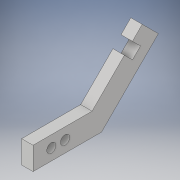
# Autodesk Inventor part: arm
Saved by Autodesk Inventor 2019 (Build 230136000, 136)
## iProperties
Created: 2018-09-08
Part Number: arm
Material: Generic
Document SubType Name: Modeling
Designer: mspet
Density: 1 g/cm^3
Appearance: Default
Author: mspet
Autodesk Inventor part; units mm, degrees
ref_plane "YZ Plane" through (0, 0, 0) normal (1, 0, 0) x (0, 1, 0)
ref_plane "XZ Plane" through (0, 0, 0) normal (0, 1, 0) x (-1, 0, 0)
ref_plane "XY Plane" through (0, 0, 0) normal (0, 0, 1) x (1, 0, 0)
sketch "Sketch1" plane through (0, 0, 0) normal (1, 0, 0) x (0, 1, 0)
  line L0 (0, 0) -> (6.35, 0)
  line L1 (6.35, 0) -> (6.35, -16.4197)
  line L2 (0, -19.05) -> (0, 0)
  circle A0 centre (3.175, -5.08) radius 1.27
  circle A1 centre (3.175, -8.89) radius 1.27
  line L3 (0, -19.05) -> (15.8114, -34.8614)
  line L4 (8.4654, -18.5351) -> (6.35, -16.4197)
  line L5 (20.3015, -30.3713) -> (19.179, -31.4938)
  line L6 (16.9339, -33.7389) -> (15.8114, -34.8614)
  line L7 (19.179, -31.4938) -> (16.9339, -33.7389)
  line L8 (15.3303, -25.4) -> (13.0852, -27.6451)
  line L9 (13.0852, -27.6451) -> (15.3303, -29.8901)
  line L10 (15.3303, -29.8901) -> (17.5753, -27.6451)
  line L11 (20.3015, -30.3713) -> (17.5753, -27.6451)
  line L12 (8.4654, -18.5351) -> (15.3303, -25.4)
  dimension "d0" = 2.54
  dimension "d1" = 3.81
  dimension "d2" = 2.54
  dimension "d3" = 5.08
  dimension "d4" = 6.35
  dimension "d5" = 3.175
  dimension "d6" = 135
  dimension "d14" = 3.175
  dimension "d15" = 12.7
  constraints: 26 end point, 4 perpendicular, 2 centre point, 2 parallel, 1 horizontal, 1 point on line
  measures "d0" diameter of A0
  measures "d1" distance of A0.centre A1.centre
  measures "d2" diameter of A1
  measures "d3" distance from line of L0 A0.centre
  measures "d4" distance of L0.start L0.end
  measures "d5" distance from line of L2 A0.centre
  measures "d6" angle of L2 L3
  measures "d14" distance between parallel lines of L10 L8
  measures "d15" distance from line of L1.end L8
extrude "Extrusion1" add sketch "Sketch1" along normal blind 3.175
body "Solid1"
